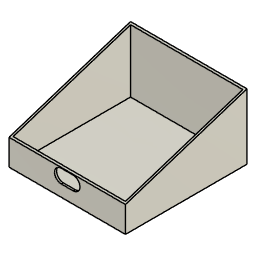
xbox-elite-s2-controller-holder v2 (Autodesk Fusion 360 design; units mm, degrees)
Autodesk Fusion 360 part; units mm, degrees
sketch "Sketch1" plane through (0, 0, 0) normal (0, 0, 1) x (1, 0, 0)
  line L0 (-95, 25) -> (-38, 25)
  line L1 (-38, 25) -> (-38, 84.5)
  line L2 (-38, 84.5) -> (-95, 84.5)
  line L3 (-95, 84.5) -> (-95, 25)
  dimension "d1" = 57
  dimension "d2" = 59.5
  constraint horizontal L0
  constraint vertical L1
  constraint horizontal L2
  constraint vertical L3
  measures "d1" distance of L0.start L0.end
  measures "d2" distance of L0.start L2.end
extrude "Extrude1" add sketch "Sketch1" along normal blind 32
shell "Shell1" thickness 1 removed faces 1 at (-76, 64.6667, 32)
draft "Draft1" angle -18 neutral plane through (-38, 84.5, 0) pull (0, 1, 0) 1 faces at (-94.6667, 64.3333, 32)
sketch "Sketch4" plane through (0, 25, 0) normal (0, -1, 0) x (1, 0, 0)
  line L0 (-95, 0) -> (-38, 0)
  line L1 (-38, 0) -> (-38, 12.6673)
  line L2 (-38, 12.6673) -> (-95, 12.6673)
  line L3 (-95, 12.6673) -> (-95, 0)
  line L4 (-63.6, 12.35) -> (-69.4, 12.35)
  arc A0 (-69.4, 12.35) -> (-69.4, 5.65) centre (-69.4, 9) ccw
  line L5 (-69.4, 5.65) -> (-63.6, 5.65)
  arc A1 (-63.6, 5.65) -> (-63.6, 12.35) centre (-63.6, 9) ccw
  line L6 (-60.25, 9) -> (-72.75, 9) construction
  dimension "d15" = 12.5
  dimension "d16" = 6.7
  constraint tangent L4 A0
  constraint tangent A0 L5
  constraint parallel L4 L5
  constraint tangent L5 A1
  constraint tangent L4 A1
  constraint midpoint A1 L6.start
  constraint midpoint A0 L6.end
  constraint horizontal L6
  measures "d15" distance of L6.start L6.end
  measures "d16" diameter of A0
extrude "Extrude4" cut sketch "Sketch4" against normal blind 1 contours L4 A0 L5 A1
